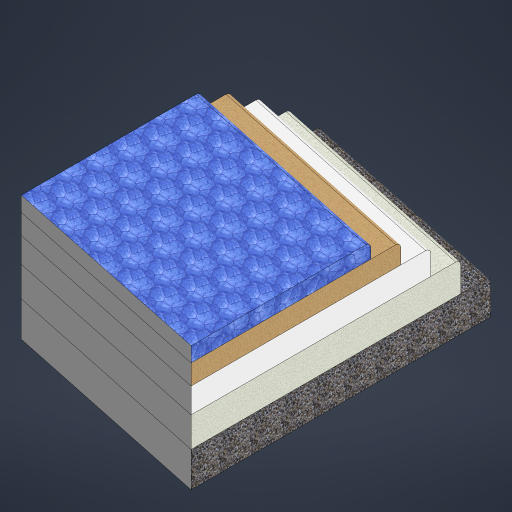
# Autodesk Inventor part: 부품1
Saved by Autodesk Inventor 2024 (Build 280153000, 153)
## iProperties
Created: 2024-01-19
Part Number: 부품1
Material: 일반
Document SubType Name: Modeling
Designer: KBU
Density: 1 g/cm^3
Appearance: 기본값
Author: KBU
Autodesk Inventor part; units mm, degrees
ref_plane "YZ Plane" through (0, 0, 0) normal (1, 0, 0) x (0, 1, 0)
ref_plane "XZ Plane" through (0, 0, 0) normal (0, 1, 0) x (-1, 0, 0)
ref_plane "XY Plane" through (0, 0, 0) normal (0, 0, 1) x (1, 0, 0)
sketch "스케치8" plane through (0, 0, 0) normal (0, 0, 1) x (1, 0, 0)
  line L0 (0, 0) -> (0, 175)
  line L1 (0, 175) -> (-850, 402.7568)
  line L2 (-850, 402.7568) -> (-850, 227.7568)
  line L3 (-850, 227.7568) -> (0, 0)
  line L4 (-40.1649, 0) -> (36.8005, 0)
  line L5 (-850, 402.7568) -> (-850, 852.7568)
  line L6 (-850, 852.7568) -> (0, 625)
  line L7 (0, 625) -> (0, 175)
  line L8 (-850, 552.7568) -> (0, 325)
  line L9 (0, 450) -> (-850, 677.7568)
  line L10 (-850, 777.7568) -> (0, 550)
  dimension "d23" = 15
  dimension "d24" = 850
  dimension "d26" = 150
  dimension "d27" = 125
  dimension "d28" = 100
  dimension "d40" = 175
  dimension "d47" = 75
  constraints: 22 end point, 7 parallel, 6 point on line, 2 horizontal, 2 vertical
  measures "d23" angle of L3 L4
  measures "d24" distance between parallel lines of L0 L2
  measures "d26" distance of L1.end L8.start
  measures "d27" distance of L9.end L8.start
  measures "d28" distance of L10.start L9.end
  measures "d40" distance of L1.end L2.end
  measures "d47" distance of L10.start L5.end
extrude "돌출9" add sketch "스케치8" against normal blind 1500 contours L3 L2 L1 L0
extrude "돌출10" add sketch "스케치8" against normal blind 1350 separate body contours L1 L5 L8 L7
extrude "돌출11" add sketch "스케치8" against normal blind 1200 separate body contours L8 L5 L9 L7
extrude "돌출12" add sketch "스케치8" against normal blind 1050 separate body contours L9 L5 L10 L7
extrude "돌출13" add sketch "스케치8" against normal blind 900 separate body contours L10 L5 L6 L7
fillet "모깎기2" radius 25 5 edges at (-425, 288.8784, -1500) (-425, 438.8784, -1350) (-425, 563.8784, -1200) (-425, 663.8784, -1050) (-425, 738.8784, -900)
